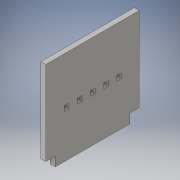
# Autodesk Inventor part: frame_front
Saved by Autodesk Inventor 2016 (Build 200138000, 138)
## iProperties
Created: 2017-09-22
Part Number: frame_front
Material: Generic
Document SubType Name: Modeling
Designer: Student
Density: 1 g/cm^3
Appearance: Default
Author: Student
Autodesk Inventor part; units mm, degrees
ref_plane "YZ Plane" through (0, 0, 0) normal (1, 0, 0) x (0, 1, 0)
ref_plane "XZ Plane" through (0, 0, 0) normal (0, 1, 0) x (-1, 0, 0)
ref_plane "XY Plane" through (0, 0, 0) normal (0, 0, 1) x (1, 0, 0)
sketch "Sketch1" plane through (0, 0, 0) normal (1, 0, 0) x (0, 1, 0)
  line L0 (7.62, 0) -> (76.2, 0)
  line L1 (76.2, 0) -> (76.2, -76.2)
  line L2 (76.2, -76.2) -> (7.62, -76.2)
  line L3 (0, -76.2) -> (0, 0) construction
  line L4 (39.5242, -14.986) -> (35.5872, -14.986)
  line L5 (35.5872, -14.986) -> (35.5872, -18.796)
  line L6 (35.5872, -18.796) -> (39.5242, -18.796)
  line L7 (39.5242, -18.796) -> (39.5242, -14.986)
  line L8 (39.5242, -25.7048) -> (35.5872, -25.7048)
  line L9 (35.5872, -25.7048) -> (35.5872, -29.5148)
  line L10 (35.5872, -29.5148) -> (39.5242, -29.5148)
  line L11 (39.5242, -29.5148) -> (39.5242, -25.7048)
  line L12 (39.5242, -36.4236) -> (35.5872, -36.4236)
  line L13 (35.5872, -36.4236) -> (35.5872, -40.2336)
  line L14 (35.5872, -40.2336) -> (39.5242, -40.2336)
  line L15 (39.5242, -40.2336) -> (39.5242, -36.4236)
  line L16 (39.5242, -47.1424) -> (35.5872, -47.1424)
  line L17 (35.5872, -47.1424) -> (35.5872, -50.9524)
  line L18 (35.5872, -50.9524) -> (39.5242, -50.9524)
  line L19 (39.5242, -50.9524) -> (39.5242, -47.1424)
  line L20 (39.5242, -57.8612) -> (35.5872, -57.8612)
  line L21 (35.5872, -57.8612) -> (35.5872, -61.6712)
  line L22 (35.5872, -61.6712) -> (39.5242, -61.6712)
  line L23 (39.5242, -61.6712) -> (39.5242, -57.8612)
  line L24 (0, -7.62) -> (7.62, -7.62)
  line L25 (7.62, -7.62) -> (7.62, 0)
  line L26 (0, -68.58) -> (7.62, -68.58)
  line L27 (7.62, -68.58) -> (7.62, -76.2)
  line L28 (0, -7.62) -> (0, -68.58)
  dimension "d8" = 12.7
  dimension "d18" = 10.6045
  dimension "d5" = 3.81
  dimension "d15" = 3.937
  dimension "d27" = 10.7188
  constraints: 58 end point, 4 parallel, 4 point on line, 3 perpendicular, 3 vertical, 2 horizontal, 1 collinear, 32 other
  measures "d5" distance of L5.end L4.end
  measures "d15" distance of L4.start L4.end
  measures "d27" distance of L4.start L8.start
extrude "Extrusion1" add sketch "Sketch1" along normal blind 4.064
body "Solid1"
